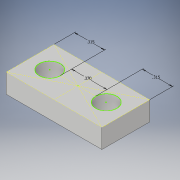
# Autodesk Inventor part: Rectangular Top Washer v1.2
Saved by Autodesk Inventor 2019 (Build 230136000, 136)
## iProperties
Created: 2020-01-11
Part Number: Rectangular Top Washer v1.2
Material: Generic
Document SubType Name: Modeling
Designer: Obscure_Decision
Density: 1 g/cm^3
Appearance: Default
Author: Obscure_Decision
Autodesk Inventor part; units mm, degrees
ref_plane "YZ Plane" through (0, 0, 0) normal (1, 0, 0) x (0, 1, 0)
ref_plane "XZ Plane" through (0, 0, 0) normal (0, 1, 0) x (-1, 0, 0)
ref_plane "XY Plane" through (0, 0, 0) normal (0, 0, 1) x (1, 0, 0)
sketch "Spacer 2D" plane through (0, 0, 0) normal (0, 1, 0) x (-1, 0, 0)
  line L0 (0, -6.35) -> (26.162, -6.35) construction
  line L1 (13.0671, 0) -> (13.0671, -12.7) construction
  line L2 (25.7671, -12.7) -> (0.3671, -12.7)
  line L3 (0.3671, -12.7) -> (0.3671, 0)
  line L4 (0.3671, 0) -> (25.7671, 0)
  line L5 (25.7671, 0) -> (25.7671, -12.7)
  line L6 (25.7671, -12.7) -> (0.3671, 0) construction
  line L7 (0.3671, -12.7) -> (25.7671, 0) construction
  line L8 (13.081, -12.7) -> (13.081, 0) construction
  line L9 (25.7949, -12.7) -> (25.7949, 0) construction
  line L10 (17.78, -6.35) -> (24.8285, -6.35) construction
  line L11 (17.78, -6.35) -> (23.368, -6.35) construction
  circle A0 centre (20.574, -6.35) radius 2.794
  circle A1 centre (5.588, -6.35) radius 2.794
  line L12 (8.382, -6.35) -> (17.78, -6.35) construction
  line L13 (0.3949, 0) -> (0.3949, -12.7) construction
  line L14 (0.381, -12.7) -> (25.781, -12.7) construction
  line L15 (25.781, -12.7) -> (25.781, 0) construction
  line L16 (25.781, 0) -> (0.381, 0) construction
  line L17 (0.381, 0) -> (0.381, -12.7) construction
  line L18 (0.381, -12.7) -> (25.781, 0) construction
  line L19 (25.781, -12.7) -> (0.381, 0) construction
  point P0 (0, 0)
  point P1 (13.0671, -6.35)
  point P2 (13.081, -6.35)
  dimension "d17" = 25.4
  dimension "d18" = 12.7
  dimension "d31" = 5.588
  dimension "d32" = 9.398
  dimension "d33" = 8.001
  dimension "d34" = 8.001
  dimension "d35" = 2.4269
  dimension "d36" = 2.4269
  constraints: 40 end point, 7 midpoint, 4 parallel, 3 horizontal, 2 horizontal alignment, 2 perpendicular, 1 point on line, 1 symmetric about line, 1 vertical, 4 other
  measures "d17" distance of L3.end L4.end
  measures "d18" distance of L4.end L2.start
  measures "d31" distance of L10.start L11.end
  measures "d32" distance of L12.start L10.start
  measures "d33" distance from line of L17 L12.start
  measures "d34" distance from line of L15 L10.start
  measures "d35" distance from line of L11.end L9
extrude "Spacer Body" add sketch "Spacer 2D" along normal blind 5.08 contours L2 L3 L4 L5 | A0 | A1
sketch "Spacer Circles" plane through (0, 5.08, 0) normal (0, 1, 0) x (1, 0, 0)
  line L0 (-13.0949, 0) -> (-13.0949, 12.7) construction
  line L1 (-0.3671, 0) -> (-0.3671, 12.7) construction
  circle A0 centre (-5.6019, 6.35) radius 2.794
  circle A1 centre (-20.5879, 6.35) radius 2.794
  line L2 (-17.7939, 6.35) -> (-8.3959, 6.35) construction
  line L3 (-25.7671, 12.7) -> (-25.7671, 0) construction
  line L4 (-25.7949, 0) -> (-0.3949, 0) construction
  line L5 (-0.3949, 0) -> (-0.3949, 12.7) construction
  line L6 (-0.3949, 12.7) -> (-25.7949, 12.7) construction
  line L7 (-25.7949, 12.7) -> (-25.7949, 0) construction
  line L8 (-25.7949, 0) -> (-0.3949, 12.7) construction
  line L9 (-0.3949, 0) -> (-25.7949, 12.7) construction
  point P0 (-13.0949, 6.35)
  dimension "d26" = 9.398
  dimension "d29" = 8.001
  dimension "d30" = 8.001
  constraints: 16 end point, 3 midpoint, 2 horizontal, 2 horizontal alignment, 2 parallel, 1 perpendicular, 1 symmetric about line, 1 vertical, 4 other
  measures "d26" distance of L2.start L2.end
  measures "d29" distance from line of L7 L2.start
  measures "d30" distance from line of L5 L2.end
extrude "Spacer Holes" cut sketch "Spacer Circles" against normal blind 10.16
equation "\"d36\" = d35"
body "Solid1"
